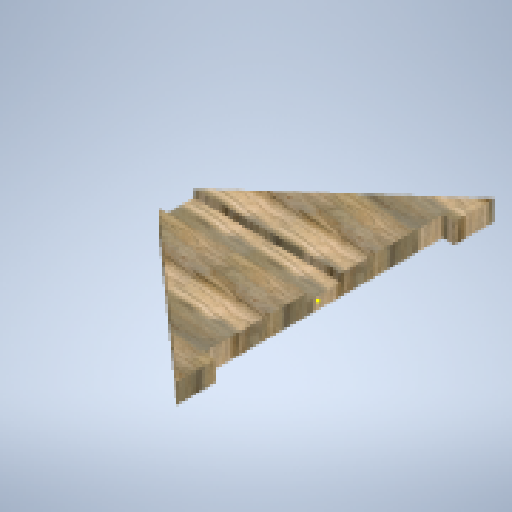
# Autodesk Inventor part: escuadra
Saved by Autodesk Inventor 2023 (Build 270158000, 158)
## iProperties
Created: 2023-03-27
Part Number: escuadra
Material: Generic
Document SubType Name: Modeling
Designer: sebas
Density: 1 g/cm^3
Appearance: Driftwood
Author: sebas
Autodesk Inventor part; units mm, degrees
ref_plane "YZ Plane" through (0, 0, 0) normal (1, 0, 0) x (0, 1, 0)
ref_plane "XZ Plane" through (0, 0, 0) normal (0, 1, 0) x (-1, 0, 0)
ref_plane "XY Plane" through (0, 0, 0) normal (0, 0, 1) x (1, 0, 0)
sketch "Sketch1" plane through (0, 0, 0) normal (0, 1, 0) x (-1, 0, 0)
  line L0 (0, 0) -> (200, 0)
  line L1 (200, 0) -> (200, -44)
  line L2 (200, -44) -> (0, -44)
  line L3 (0, -44) -> (0, 0)
  line L4 (0, -22) -> (0, -222)
  line L5 (0, -222) -> (200, -44)
  line L6 (0, -22) -> (0, 178)
  line L7 (0, 178) -> (200, 0)
  dimension "d0" = 200
  dimension "d1" = 44
  dimension "d2" = 200
  dimension "d3" = 200
  constraints: 16 end point, 2 perpendicular, 2 vertical, 1 horizontal, 1 midpoint, 1 point on line
  measures "d0" distance of L0.start L0.end
  measures "d1" distance of L0.end L1.end
  measures "d2" distance of L4.start L4.end
  measures "d3" distance of L4.start L6.end
extrude "Extrusion1" add sketch "Sketch1" along normal blind 25.4
sketch "Sketch2" plane through (0, 25.4, 0) normal (0, 1, 0) x (1, 0, 0)
  line L0 (-200, 0) -> (0, -178) projected
  line L1 (-200, 0) -> (0, 0)
  line L2 (0, -178) -> (0, 222) projected
  line L3 (0, 222) -> (-200, 44) projected
  line L4 (-200, 44) -> (0, 44)
  line L5 (0, 0) -> (0, 44)
  line L6 (-200, 44) -> (-200, 0) projected
  line L7 (-200, 0) -> (-200, 44)
  constraints: 8 end point, 2 collinear, 2 perpendicular, 1 point on line
sketch "Sketch3" plane through (0, 25.4, 0) normal (0, 1, 0) x (1, 0, 0)
  point P0 (0, 0)
extrude "Extrusion2" cut sketch "Sketch2" against normal blind 10 contours L6 L4 L2 L1
sketch "Sketch4" plane through (0, 25.4, 0) normal (0, 1, 0) x (1, 0, 0)
  line L0 (0, -128) -> (-15, -128)
  line L1 (0, 222) -> (-200, 44) projected
  line L2 (0, 44) -> (0, 222) projected
  line L3 (0, 172) -> (-15, 172)
  line L4 (-15, 172) -> (-15, -128)
  line L5 (-200, 44) -> (0, 44) projected
  line L6 (0, -128) -> (0, 172)
  point P0 (0, 0)
  point P1 (0, -178)
  dimension "d8" = 50
  dimension "d10" = 50
  constraints: 8 end point, 1 horizontal, 1 perpendicular, 1 point on line
  measures "d8" distance of point (0, -178) L0.start
  measures "d10" distance of L1.start L3.start
extrude "Extrusion3" cut sketch "Sketch4" against normal through all contours L0 L4 L5 L6 | L5 L4 L3 L2
body "Solid1"
